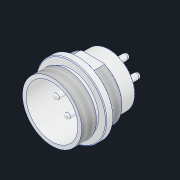
# Autodesk Inventor part: PLT-164-R-R
Saved by Autodesk Inventor 2021 (Build 250183000, 183)
## iProperties
Created: 2021-07-21
Part Number: PLT-164-R-R
Material: アルミニウム 6061
Document SubType Name: Modeling
Designer: yuta0
Density: 2.7 g/cm^3
Appearance: アルミニウム - フラット
Author: yuta0
Autodesk Inventor part; units mm, degrees
ref_plane "YZ Plane" through (0, 0, 0) normal (1, 0, 0) x (0, 1, 0)
ref_plane "XZ Plane" through (0, 0, 0) normal (0, 1, 0) x (-1, 0, 0)
ref_plane "XY Plane" through (0, 0, 0) normal (0, 0, 1) x (1, 0, 0)
sketch "スケッチ1" plane through (0, 0, 0) normal (1, 0, 0) x (0, 1, 0)
  line L0 (0, 0) -> (8, 0)
  line L1 (8, 0) -> (8, -4)
  line L2 (8, -4) -> (7.5, -4)
  line L3 (7.5, -4) -> (7.5, -5.1)
  line L4 (7.5, -5.1) -> (9.5, -5.1)
  line L5 (9.5, -5.1) -> (9.5, -7.1)
  line L6 (9.5, -7.1) -> (8, -7.1)
  line L7 (7, -15.5) -> (0, -15.5)
  line L8 (0, -15.5) -> (0, 0)
  line L9 (7, 0) -> (7, -10)
  line L10 (7, -10) -> (0, -10)
  line L11 (8, -7.1) -> (8, -11.1)
  line L12 (8, -11.1) -> (7, -11.1)
  line L13 (7, -11.1) -> (7, -15.5)
  dimension "d0" = 8
  dimension "d1" = 9.5
  dimension "d3" = 5.1
  dimension "d4" = 2
  dimension "d5" = 15.5
  dimension "d6" = 0.5
  dimension "d7" = 4
  dimension "d8" = 7
  dimension "d9" = 10
  dimension "d13" = 4
  dimension "d14" = 8
  dimension "d15" = 1
  constraints: 28 end point, 9 perpendicular, 2 horizontal, 2 point on line, 2 vertical
  measures "d0" distance between parallel lines of L8 L1
  measures "d1" distance between parallel lines of L8 L5
  measures "d3" distance between parallel lines of L0 L4
  measures "d4" distance of L4.end L5.end
  measures "d5" distance between parallel lines of L7 L0
  measures "d6" distance of L1.end L2.end
  measures "d7" distance of L0.end L1.end
  measures "d8" distance between parallel lines of L8 L9
  measures "d9" distance of L9.start L9.end
  measures "d13" distance of L6.end L11.end
  measures "d14" distance between parallel lines of L8 L11
  measures "d15" distance of L11.end L12.end
revolve "回転1" add sketch "スケッチ1" angle 360 about axis through (0, 0, -15.5) along (0, 0, 1) contours L0 L1 L2 L3 L4 L5 L6 L11 L12 L13 L7 L8 L10 L9
thread "ねじ1" size "M16x2" class "6g" standard "ANSI Metric M Profile" length 12
thread "ねじ2" size "M16x2" class "6g" standard "ANSI Metric M Profile" length 12
fillet "フィレット1" radius 0.2 5 edges at (0, -9.5, -5.1) (0, -9.5, -7.1) (0, -7, -15.5) (0, -7, -11.1) (0, -8, -11.1)
sketch "スケッチ2" plane through (0, 0, -11.1) normal (0, 0, -1) x (-1, 0, 0)
  circle A0 centre (0, 0) radius 8 projected
  line L0 (3.2726, 7.3) -> (-3.2726, 7.3)
  dimension "d19" = 7.3
  constraints: 2 end point, 2 point on circle, 1 horizontal
  measures "d19" distance from line of point (0, 0) L0
extrude "押し出し1" cut sketch "スケッチ2" against normal up to surface (4 mm away) contours L0 A0 picked at (0, 7.5333)
sketch "スケッチ3" plane through (0, 0, -15.5) normal (0, 0, -1) x (-1, 0, 0)
  circle A0 centre (-3, 0) radius 0.75
  circle A1 centre (3, 0) radius 0.75
  point P0 (0, 0)
  dimension "d22" = 1.5
  dimension "d23" = 1.5
  dimension "d24" = 3
  dimension "d25" = 3
  constraints: 2 centre point, 2 horizontal alignment
  measures "d22" diameter of A0
  measures "d23" diameter of A1
  measures "d24" distance of point (0, 0) A0.centre
  measures "d25" distance of point (0, 0) A1.centre
extrude "押し出し2" add sketch "スケッチ3" along normal blind 5 and the other way blind 12
fillet "フィレット2" radius 0.75 4 edges at (-2.25, 0, -3.5) (3.75, 0, -3.5) (-2.25, 0, -20.5) (3.75, 0, -20.5)
pattern_circular "円形状パターン1" count 4 over 360 about axis through (0, 0, -10) along (0, 0, 1) of "押し出し2", "フィレット2"
